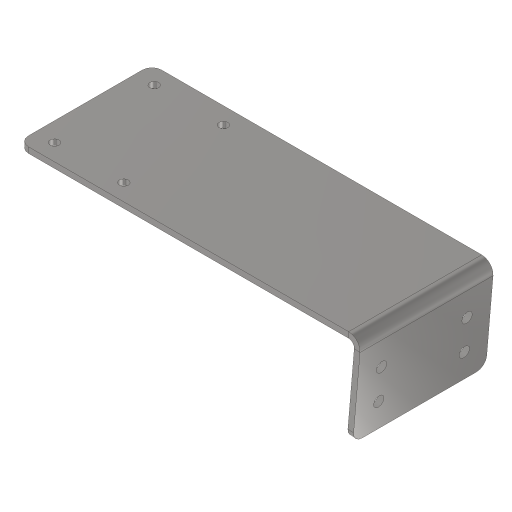
# Autodesk Inventor part: 26062025_2
Saved by Autodesk Inventor 2024.3 (Build 283343000, 343)
## iProperties
Created: 2025-06-26
Part Number: 26062025_2
Material: AISI 304
Document SubType Name: Sheet Metal
Designer: PM
Density: 8 g/cm^3
Sheet Metal Rule: Default_mm
Appearance: Semi-Polished
Flat Pattern Width: 7 cm
Flat Pattern Length: 22.4067 cm
Flat Pattern Area: 156.847 cm^2
Sheet Metal Width: 70,000 mm
Sheet Metal Length: 224,067 mm
Sheet Metal Area: 15684,699 mm^2
Description: Uchwyt_ZPP
Mass: 372.401 g
Surface Area: 331.622 cm^2
Volume: 46.5501 cm^3
Author: PM
Revision Number: 00
Autodesk Inventor part; units mm, degrees
ref_plane "YZ Plane" through (0, 0, 0) normal (1, 0, 0) x (0, 1, 0)
ref_plane "XZ Plane" through (0, 0, 0) normal (0, 1, 0) x (-1, 0, 0)
ref_plane "XY Plane" through (0, 0, 0) normal (0, 0, 1) x (1, 0, 0)
sketch "Sketch1" plane through (0, 0, 0) normal (0, 1, 0) x (-1, 0, 0)
  line L0 (-90, 35) -> (90, 35)
  line L1 (90, 35) -> (90, -35)
  line L2 (90, -35) -> (-90, -35)
  line L3 (-90, -35) -> (-90, 35)
  line L4 (-90, 35) -> (90, -35) construction
  line L5 (90, 35) -> (-90, -35) construction
  point P0 (0, 0)
  dimension "d0" = 70
  dimension "d1" = 180
  measures "d0" distance of L0.end L1.end
  measures "d1" distance of L1.end L2.end
extrude "Plate1" add sketch "Sketch1" along normal blind 3
sketch "Sketch2" plane through (87.0114, 3.2615, 35) normal (0.9961947, -0.0871557, 0) x (0.0871557, 0.9961947, 0)
  line L0 (0, -70) -> (0, 0)
  line L1 (0, 0) -> (-50, 0)
  line L2 (-50, 0) -> (-50, -70)
  line L3 (-50, -70) -> (0, -70)
  constraints: 6 end point, 1 horizontal, 1 perpendicular, 1 vertical
edge flange "Flange1" height 50 angle 95 thickness 3 bend radius 3 thickness toward (0.9961947, -0.0871557, 0) relief tear relief width 3 relief depth 1.5 edges at (90, 0, 0) wall of the first edge with corners at (87.0114, 3.2615, -35) (87.0114, 3.2615, 35) (82.6536, -46.5483, 35) (82.6536, -46.5483, -35)
bend "Bend1"
corner "Corner1"
sketch "Sketch3" plane through (0, 3, 0) normal (0, 1, 0) x (1, 0, 0)
  line L0 (-43.6, -26.2) -> (-80, -26.2) construction
  line L1 (-80, -26.2) -> (-80, 26.2) construction
  line L2 (-80, 26.2) -> (-43.6, 26.2) construction
  line L3 (-43.6, 26.2) -> (-43.6, -26.2) construction
  line L4 (-43.6, -26.2) -> (-80, 26.2) construction
  line L5 (-80, -26.2) -> (-43.6, 26.2) construction
  line L6 (-90, -35) -> (-90, 35) construction
  point P0 (0, 0)
  point P1 (-61.8, 0)
  dimension "d13" = 52.4
  dimension "d14" = 36.4
  dimension "d15" = 10
  constraints: 12 end point, 4 coincident, 2 midpoint, 2 parallel, 1 horizontal, 1 horizontal alignment, 1 perpendicular
  measures "d13" distance of L0.end L1.end
  measures "d14" distance of L1.end L2.end
  measures "d15" distance between parallel lines of L6 L1
hole "Hole1" at (-80, 3, 26.2) at (-80, 3, -26.2) at (-43.6, 3, -26.2) at (-43.6, 3, 26.2) direction (0, -1, 0) diameter 4.8 end through all clearance for "Countersunk Flat Head Screw DIN EN ISO 2009" size "M4" standard "DIN"
sketch "Sketch4" plane through (82.6536, -46.5483, -35) normal (-0.9961947, 0.0871557, 0) x (0, 0, 1)
  line L0 (12.5, 13.5) -> (57.5, 13.5) construction
  line L1 (57.5, 13.5) -> (57.5, 29.9521) construction
  line L2 (57.5, 29.9521) -> (12.5, 29.9521) construction
  line L3 (12.5, 29.9521) -> (12.5, 13.5) construction
  line L4 (12.5, 13.5) -> (57.5, 29.9521) construction
  line L5 (57.5, 13.5) -> (12.5, 29.9521) construction
  line L6 (70, 43.4521) -> (0, 43.4521) construction
  line L7 (0, 43.4521) -> (0, 0) construction
  line L8 (0, 0) -> (70, 0) construction
  line L9 (70, 43.4521) -> (70, 0) construction
  circle A0 centre (57.5, 29.9521) radius 2.75
  line L10 (53.5346, 32.7021) -> (62.0591, 32.7021)
  point P0 (35, 39.1674)
  point P1 (35, 21.7261)
  point P2 (70, 21.7261)
  dimension "d23" = 0
  dimension "d24" = 70
  dimension "d25" = 45
  dimension "d26" = 13.5
  dimension "d27" = 16.4521
  dimension "d28" = 5.5
  dimension "d29" = 10.75
  constraints: 14 end point, 5 coincident, 3 midpoint, 3 parallel, 1 centre point, 1 horizontal, 1 perpendicular, 1 tangent, 1 vertical alignment
  measures "d23" vertical distance of point (70, 21.726) point (35, 21.726)
  measures "d24" distance of L7.end L8.end
  measures "d25" distance of L0.start L0.end
  measures "d26" distance between parallel lines of L8 L0
  measures "d27" distance of L2.end L0.start
  measures "d28" diameter of A0
  measures "d29" distance between parallel lines of L6 L10
hole "Hole2" at (85.2641, -16.7101, -22.5) at (83.8302, -33.0996, -22.5) at (85.2641, -16.7101, 22.5) at (83.8302, -33.0996, 22.5) direction (0.9961947, -0.0871557, 0) diameter 5.5 end through all clearance for "Countersunk Flat Head Screw DIN EN ISO 2009" size "M5" standard "DIN"
fillet "Fillet1" radius 5 4 edges at (84.1479, -46.679, 35) (84.1479, -46.679, -35) (-90, 1.5, 35) (-90, 1.5, -35)
equation "\"d21\" = Thickness"
equation "\"d35\" = Thickness"
equation "\"d2\" = Thickness"
equation "\"d3\" = BendReliefWidth"
equation "\"d4\" = BendReliefDepth"
equation "\"d5\" = MinimumRemnant"
equation "\"d6\" = TransitionRadius"
equation "\"d9\" = BendRadius"
equation "\"d10\" = CornerReliefSize"
equation "\"d11\" = GapSize"
equation "\"d12\" = JacobiRadiusSize"
equation "\"BendRadius\" = Thickness"
equation "\"BendReliefWidth\" = Thickness"
equation "\"BendReliefDepth\" = 0.5 * Thickness"
equation "\"CornerReliefSize\" = 4 * Thickness"
equation "\"MinimumRemnant\" = 2 * Thickness"
equation "\"TransitionRadius\" = BendRadius"
equation "\"JacobiRadiusSize\" = BendRadius"
equation "\"GapSize\" = Thickness"
equation "\"Thickness\" = 3"
body "Solid1"
